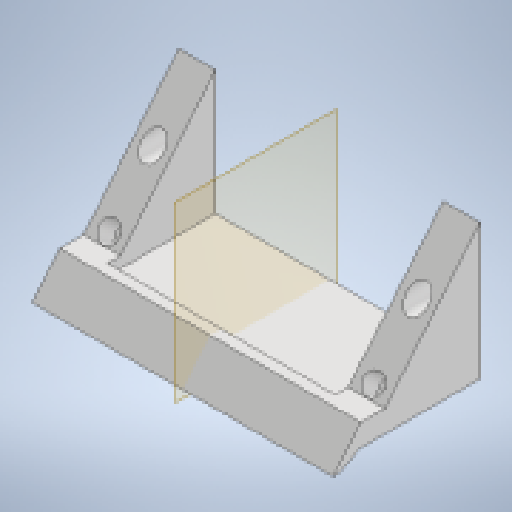
# Autodesk Inventor part: MS_podstawa
Saved by Autodesk Inventor 2023 (Build 270158000, 158)
## iProperties
Created: 2024-04-29
Part Number: MS_podstawa
Material: Ogólny
Document SubType Name: Modeling
Designer: kamil
Density: 1 g/cm^3
Appearance: Domyślna
Author: kamil
Autodesk Inventor part; units mm, degrees
ref_plane "YZ Plane" through (0, 0, 0) normal (1, 0, 0) x (0, 1, 0)
ref_plane "XZ Plane" through (0, 0, 0) normal (0, 1, 0) x (-1, 0, 0)
ref_plane "XY Plane" through (0, 0, 0) normal (0, 0, 1) x (1, 0, 0)
sketch "Szkic1" plane through (0, 0, 0) normal (0, 1, 0) x (-1, 0, 0)
  line L0 (9.0922, 8.517) -> (-72.9078, 8.517)
  line L1 (-72.9078, 8.517) -> (-72.9078, -31.483)
  line L2 (-72.9078, -31.483) -> (9.0922, -31.483)
  line L3 (9.0922, -31.483) -> (9.0922, 8.517)
  point P0 (0, 0)
  dimension "d0" = 82
  dimension "d1" = 40
  constraints: 8 end point, 2 parallel, 1 horizontal, 1 perpendicular
  measures "d0" distance of L2.end L1.end
  measures "d1" distance of L1.end L0.end
extrude "Wyciągnięcie proste1" add sketch "Szkic1" along normal blind 2
sketch "Szkic2" plane through (-9.0922, 0, -31.483) normal (-1, 0, 0) x (0, 0, 1)
  line L0 (40, 0) -> (40, 2) projected
  line L1 (0, 0) -> (40, 0) projected
  line L2 (0, 0) -> (40, 0) projected
  line L3 (40, 0) -> (40, 2) projected
  line L4 (0, 2) -> (40, 2) projected
  line L5 (0, 0) -> (0, 2) projected
  line L6 (40, -3) -> (35.8045, 2)
  line L7 (40, -3) -> (38, -3)
  line L8 (38, -3) -> (29.3397, 2)
  line L9 (40, 2) -> (0, 2) projected
  point P0 (31.483, 0)
  point P1 (40, 1)
  point P2 (37.4827, 0)
  point P3 (32.8038, 0)
  dimension "d4" = 3
  dimension "d5" = 50
  dimension "d6" = 2
  dimension "d11" = 150
  constraints: 6 end point, 2 point on line, 1 horizontal, 1 midpoint, 1 vertical alignment
  measures "d4" distance from line of L6.start L1
  measures "d5" angle of L4 L6
  measures "d6" distance of L6.start L7.end
  measures "d11" angle of L7 L8
extrude "Wyciągnięcie proste2" cut sketch "Szkic2" against normal through all contours L1 L6 L4 L0
extrude "Wyciągnięcie proste3" add sketch "Szkic2" against normal up to surface (82 mm away) contours L6 L7 L8 L1
sketch "Szkic4" plane through (-9.0922, 0, -31.483) normal (-1, 0, 0) x (0, 0, 1)
  line L0 (0, 0) -> (0, 2) projected
  line L1 (40, -3) -> (35.8045, 2) projected
  line L2 (40, -3) -> (35.8045, 2)
  line L3 (35.8045, 2) -> (0, 44.6701)
  line L4 (35.8045, 2) -> (0, 2) projected
  line L5 (0, 2) -> (0, 44.6701)
  point P0 (31.483, 0)
  constraints: 6 end point, 2 collinear, 1 vertical
extrude "Wyciągnięcie proste5" add sketch "Szkic4" against normal blind 10
sketch "Szkic5" plane through (-9.0922, 0, -31.483) normal (-1, 0, 0) x (0, 0, 1)
  line L0 (40, -3) -> (0, 44.6701) projected
  line L1 (36.1698, -6.2139) -> (-3.8302, 41.4562)
  line L2 (0, 2) -> (35.8045, 2) projected
  line L3 (0, 5) -> (34.9654, 5)
  line L4 (0, 44.6701) -> (0, 36.8915)
  line L5 (0, 0) -> (0, 44.6701) projected
  point P0 (31.483, 0)
  point P1 (26.7602, 5)
  point P2 (33.2872, 5)
  dimension "d17" = 5
  dimension "d18" = 3
  constraints: 6 end point, 2 parallel, 2 point on line
  measures "d17" distance between parallel lines of L0 L1
  measures "d18" distance between parallel lines of L2 L3
extrude "Wyciągnięcie proste6" cut sketch "Szkic5" against normal through all contours L3 L1 L4 L0
sketch "Szkic6" plane through (72.9078, 0, -31.483) normal (0, 0, -1) x (-1, 0, 0)
  circle A0 centre (77, 22.5) radius 2.85 projected
  circle A1 centre (77, 22.5) radius 1.6
  circle A2 centre (77, 22.5) radius 3
  point P0 (72.9078, 0)
  dimension "d21" = 3.2
  dimension "d22" = 6
  constraints: 2 centre point, 2 coincident
  measures "d21" diameter of A1
  measures "d22" diameter of A2
extrude "Wyciągnięcie proste7" cut sketch "Szkic6" against normal through all contours A0 | A1 | A2
sketch "Szkic7" plane through (72.9078, 0, -31.483) normal (0, 0, -1) x (-1, 0, 0)
  circle A0 centre (77, 22.5) radius 3 projected
  circle A1 centre (77, 22.5) radius 1.6
  point P0 (72.9078, 0)
  dimension "d25" = 3.2
  constraints: 1 centre point, 1 coincident
  measures "d25" diameter of A1
extrude "Wyciągnięcie proste8" add sketch "Szkic7" against normal blind 5
sketch "Szkic8" plane through (-9.0922, 36.8915, -31.483) normal (0, 0.6427876, 0.7660444) x (1, 0, 0)
  ellipse E0 centre (5, -18.7868) end of major axis (5, -22.703) minor radius 3 projected
  line L0 (10, 0) -> (10, -41.6314) projected
  line L1 (0, 0) -> (10, 0) projected
  line L2 (0, -41.6314) -> (0, 0) projected
  line L3 (0, -41.6314) -> (10, -41.6314) projected
  ellipse E1 centre (5, -18.7868) end of major axis (5, -22.703) minor radius 3 construction
  point P0 (9.0922, -48.4974)
  point P1 (5, -38.6314)
  dimension "d28" = 3
  constraints: 1 vertical alignment, 2 other
  measures "d28" distance from line of L3 point (5, -38.631)
hole "Otwór1" at (-4.0922, 7.2981, -6.6512) direction (0, -0.6427876, -0.7660444) diameter 3.2 depth 14 counterbore diameter 5.7 counterbore depth 6
sketch "Szkic9" plane through (-9.0922, 0, -31.483) normal (-1, 0, 0) x (0, 0, 1)
  line L0 (26.7602, 5) -> (0, 36.8915) projected
  line L1 (0, 2) -> (35.8045, 2) projected
  line L2 (40, -3) -> (33.2872, 5) projected
  line L3 (33.2872, 5) -> (26.7602, 5) projected
  line L4 (0, 36.8915) -> (26.7602, 5) projected
  line L5 (26.7602, 5) -> (26.7602, 2)
  point P0 (31.483, 0)
  constraints: 2 end point, 1 perpendicular, 1 point on line
extrude "Wyciągnięcie proste9" add sketch "Szkic9" against normal up to surface (82 mm away)
ref_plane "Płaszczyzna konstrukcyjna1" through (31.9078, 0, -31.483) normal (1, 0, 0) x (0, 0, -1)
mirror "Odbij1" about plane through (31.9078, 0, -31.483) normal (1, 0, 0) of "Otwór1", "Wyciągnięcie proste8", "Wyciągnięcie proste7", "Wyciągnięcie proste6", "Wyciągnięcie proste5"
sketch "Szkic10" plane through (0.9078, 2, -4.7228) normal (0, 0, -1) x (-1, 0, 0)
  line L0 (-62, 3) -> (-62, 0) projected
  line L1 (0, 0) -> (-62, 0) projected
  line L2 (0, 3) -> (0, 0) projected
  line L3 (0, 3) -> (-62, 3) projected
  point P0 (0.9078, -2)
extrude "Wyciągnięcie proste10" cut sketch "Szkic10" against normal blind 3.5
sketch "Szkic13" plane through (0.9078, 0, -31.483) normal (1, 0, 0) x (0, 0, -1)
  line L0 (0, 2) -> (-30.2602, 2) projected
  line L1 (0, 2) -> (0, 36.8915) projected
  line L2 (0, 36.8915) -> (-26.7602, 5) projected
  line L3 (-30.2602, 5) -> (-26.7602, 5) projected
  line L4 (-30.2602, 5) -> (-30.2602, 2) projected
  point P0 (-31.483, 0)
extrude "Wyciągnięcie proste12" cut sketch "Szkic13" against normal blind 1.5
mirror "Odbij2" about plane through (31.9078, 0, -31.483) normal (1, 0, 0) of "Wyciągnięcie proste12"
